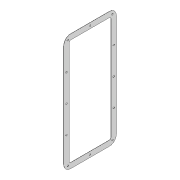
# Autodesk Inventor part: GB-gasket
Saved by Autodesk Inventor 2020 (Build 240168000, 168)
## iProperties
Created: 2021-06-24
Part Number: GB-gasket
Material: Generic
Document SubType Name: Modeling
Designer: Aidan Lee
Density: 1 g/cm^3
Appearance: Smooth - White
Author: Aidan Lee
Autodesk Inventor part; units mm, degrees
ref_plane "YZ Plane" through (0, 0, 0) normal (1, 0, 0) x (0, 1, 0)
ref_plane "XZ Plane" through (0, 0, 0) normal (0, 1, 0) x (-1, 0, 0)
ref_plane "XY Plane" through (0, 0, 0) normal (0, 0, 1) x (1, 0, 0)
sketch "Sketch1" plane through (0, 0, 0) normal (0, 0, 1) x (1, 0, 0)
  line L0 (0, 0) -> (140, 0) construction
  line L1 (140, 0) -> (140, 310) construction
  line L2 (140, 310) -> (0, 310) construction
  line L3 (0, 310) -> (0, 0) construction
  line L4 (15, 295) -> (125, 295) construction
  line L5 (125, 295) -> (125, 15) construction
  line L6 (125, 15) -> (15, 15) construction
  line L7 (15, 15) -> (15, 295) construction
  line L8 (15, 295) -> (125, 295) construction
  line L9 (70, 314.0975) -> (70, 322.6254) construction
  line L10 (15, 295) -> (15, 269.8596) construction
  line L11 (125, 295) -> (125, 292.6022) construction
  line L12 (0, 165.5) -> (-18, 165.5) construction
  line L13 (-18, 165.5) -> (-18, 185.5) construction
  line L14 (-18, 185.5) -> (0, 185.5) construction
  line L15 (0, 185.5) -> (0, 165.5) construction
  line L16 (-24.3067, 155) -> (-34.4998, 155) construction
  circle A0 centre (-9, 175.5) radius 3 construction
  line L17 (-18, 185.5) -> (0, 205.5) construction
  line L18 (0, 144.5) -> (-18, 144.5) construction
  line L19 (-18, 144.5) -> (-18, 124.5) construction
  circle A1 centre (-9, 134.5) radius 3 construction
  line L20 (-18, 124.5) -> (0, 104.5) construction
  line L21 (140, 165.5) -> (158, 165.5) construction
  line L22 (158, 165.5) -> (158, 185.5) construction
  circle A2 centre (149, 175.5) radius 3 construction
  line L23 (158, 185.5) -> (140, 205.5) construction
  line L24 (158, 144.5) -> (158, 124.5) construction
  line L25 (140, 144.5) -> (158, 144.5) construction
  circle A3 centre (149, 134.5) radius 3 construction
  line L26 (158, 124.5) -> (140, 104.5) construction
  line L27 (0, 300.2843) -> (9.7157, 310) construction
  line L28 (140, 300.2843) -> (130.2843, 310) construction
  line L29 (0, 9.7157) -> (9.7157, 0) construction
  line L30 (140, 9.7157) -> (130.2843, 0) construction
  line L31 (70, 295) -> (70, 310) construction
  line L32 (0, 155) -> (15, 155) construction
  line L33 (23.9173, 286.0827) -> (15, 295) construction
  line L34 (16.5096, 292.7523) -> (17.2477, 293.4904) construction
  line L35 (23.9173, 286.0827) -> (16.8787, 293.1213) construction
  line L36 (123.4904, 292.7523) -> (122.7523, 293.4904) construction
  line L37 (15, 17.2679) -> (15, 136.2679) construction
  arc A4 (14, 16.2679) -> (15, 17.2679) centre (14, 17.2679) ccw construction
  line L38 (14, 16.2679) -> (12, 16.2679) construction
  arc A5 (17, 17.2679) -> (18, 16.2679) centre (18, 17.2679) ccw construction
  spline S0 degree 3 poles (123.4904, 292.7523) (126.7806, 289.462) (122.6845, 284.0803) (122.5, 267.9145) knots 0 0 0 0 1 1 1 1 construction
  line L39 (15.2393, 288.9289) -> (15.2393, 218.384) construction
  line L40 (125, 148.5289) -> (125, 140.8711) construction
  line L41 (-110.1015, 148.4668) -> (-137.337, 121.2312) construction
  line L42 (-137.337, 121.2312) -> (-99.9418, 121.2312) construction
  line L43 (209.7417, 198.7679) -> (209.7417, 184.7679) construction
  line L44 (15, 148.5289) -> (15, 140.2675) construction
  line L45 (125, 148.5289) -> (125, 140.2675) construction
  spline S1 degree 4 poles (17.2477, 293.4904) (18.1955, 294.4381) (19.6714, 295.0826) (20.7017, 295) (21.8623, 295) knots 0 0 0 0 0 1 1 1 1 1 construction
  spline S2 degree 3 poles (122.7523, 293.4904) (121.4886, 294.7541) (119.4432, 295.1927) (118.1377, 295) knots 0 0 0 0 1 1 1 1 construction
  line L46 (118.1377, 295) -> (21.8623, 295) construction
  line L47 (16.8787, 293.1213) -> (23.2316, 286.7684) construction
  arc A6 (19, 310) -> (0, 291) centre (19, 291) ccw construction
  arc A7 (19, 295) -> (15, 291) centre (19, 291) ccw construction
  line L48 (19, 291) -> (10, 291) construction
  line L49 (19, 291) -> (19, 300) construction
  line L50 (16.1716, 293.8284) -> (5.565, 304.435) construction
  circle A8 centre (10.8683, 299.1317) radius 2 construction
  line L51 (9.8231, 300.915) -> (9.085, 300.1769) construction
  line L52 (11.9134, 297.3485) -> (12.6515, 298.0866) construction
  circle A9 centre (70, 302.5) radius 2 construction
  circle A10 centre (7.5, 155) radius 2 construction
  circle A11 centre (7.5, 227.0659) radius 2 construction
  line L53 (7.5, 155) -> (7.5, 227.0659) construction
  line L54 (7.5, 227.0659) -> (7.5, 299.1317) construction
  arc A12 (140, 291) -> (121, 310) centre (121, 291) ccw construction
  arc A13 (125, 291) -> (121, 295) centre (121, 291) ccw construction
  circle A14 centre (129.1317, 299.1317) radius 2 construction
  circle A15 centre (132.5, 155) radius 2 construction
  circle A16 centre (132.5, 227.0659) radius 2 construction
  circle A17 centre (10.8683, 10.8683) radius 2 construction
  circle A18 centre (70, 7.5) radius 2 construction
  circle A19 centre (7.5, 82.9341) radius 2 construction
  circle A20 centre (132.5, 82.9341) radius 2 construction
  circle A21 centre (129.1317, 10.8683) radius 2 construction
  arc A22 (0, 19) -> (19, 0) centre (19, 19) ccw construction
  arc A23 (15, 19) -> (19, 15) centre (19, 19) ccw construction
  arc A24 (121, 0) -> (140, 19) centre (121, 19) ccw construction
  arc A25 (121, 15) -> (125, 19) centre (121, 19) ccw construction
  circle A26 centre (10.8683, 299.1317) radius 7.5 construction
  line L55 (4.4716, 303.3416) -> (6.8718, 305.7419) construction
  line L56 (15, 140.2675) -> (15, 136.2679) construction
  line L57 (125, 138.6822) -> (125, 140.2675) construction
  line L58 (15, 138.6822) -> (15, 140.2675) construction
  line L59 (19, 15) -> (121, 15) construction
  line L60 (121, 0) -> (19, 0) construction
  line L61 (15, 291) -> (15, 19) construction
  line L62 (0, 19) -> (0, 291) construction
  line L63 (125, 291) -> (125, 19) construction
  line L64 (140, 19) -> (140, 291) construction
  line L65 (19, 295) -> (121, 295) construction
  line L66 (121, 310) -> (19, 310) construction
  arc A27 (132.5, 291) -> (121, 302.5) centre (121, 291) ccw construction
  arc A28 (139.5, 291) -> (121, 309.5) centre (121, 291) ccw
  arc A29 (125.5, 291) -> (121, 295.5) centre (121, 291) ccw
  arc A30 (125.5, 291) -> (139.5, 291) centre (132.5, 291) ccw construction
  arc A31 (121, 309.5) -> (121, 295.5) centre (121, 302.5) ccw construction
  arc A32 (19, 309.5) -> (0.5, 291) centre (19, 291) ccw
  arc A33 (19, 295.5) -> (14.5, 291) centre (19, 291) ccw
  arc A34 (121, 0.5) -> (139.5, 19) centre (121, 19) ccw
  arc A35 (121, 14.5) -> (125.5, 19) centre (121, 19) ccw
  arc A36 (14.5, 19) -> (19, 14.5) centre (19, 19) ccw
  arc A37 (0.5, 19) -> (19, 0.5) centre (19, 19) ccw
  line L67 (139.5, 19) -> (139.5, 291)
  line L68 (125.5, 291) -> (125.5, 19)
  line L69 (121, 14.5) -> (19, 14.5)
  line L70 (19, 0.5) -> (121, 0.5)
  line L71 (14.5, 19) -> (14.5, 291)
  line L72 (0.5, 291) -> (0.5, 19)
  line L73 (121, 295.5) -> (19, 295.5)
  line L74 (19, 309.5) -> (121, 309.5)
  point P0 (70, 318.3615)
  point P1 (-29.4032, 155)
  point P2 (-18, 175.5)
  point P3 (-9, 185.5)
  point P4 (124.7607, 288.9289)
  point P5 (209.7417, 191.7679)
  point P6 (19.6961, 294.835)
  point P7 (120.3039, 294.835)
  point P8 (9.4541, 300.5459)
  point P9 (12.2825, 297.7175)
  dimension "d163" = 4
  dimension "d0" = 140
  dimension "d1" = 310
  dimension "d2" = 15
  dimension "d85" = 18
  dimension "d86" = 20
  dimension "d87" = 10.5
  dimension "d88" = 6
  dimension "d89" = 20
  dimension "d114" = 135
  dimension "d126" = 1
  dimension "d128" = 2
  dimension "d152" = 45
  dimension "d158" = 45
  dimension "d161" = 4
  dimension "d164" = 5.5
  dimension "d168" = 15
  dimension "d169" = 1
  dimension "d170" = 1
  dimension "d171" = 1
  dimension "expansion" = 0.5
  dimension "d201" = 0.5
  constraints: 150 end point, 65 symmetric about line, 45 point on circle, 37 centre point, 16 midpoint, 16 parallel, 15 point on line, 14 tangent, 10 horizontal, 9 horizontal alignment, 9 vertical, 8 collinear, 8 perpendicular, 7 vertical alignment, 5 coincident, 3 equal length, 1 equal radius, 42 other
  measures "d0" distance of L0.start L0.end
  measures "d1" distance of L2.end L0.start
  measures "d2" distance between parallel lines of L2 L4
  measures "d85" distance of L13.end L14.end
  measures "d86" distance of L12.end L13.end
  measures "d87" distance between parallel lines of L12 L16
  measures "d88" diameter of A0
  measures "d89" vertical distance of L13.end L17.end
  measures "d114" angle of L3 L27
  measures "d126" radius of A4
  measures "d128" distance of L38.start L38.end
  measures "d152" angle of L42 L41
  measures "d158" angle of L4 L35
  measures "d161" radius of A7
  measures "d164" distance edge to line of A6 L51
  measures "d168" diameter of A26
  measures "d169" distance between parallel lines of L27 L55
  measures "d170" distance from line of L50.start L34
  measures "d171" horizontal distance between centres of A23 A5
  measures "expansion" radial gap between concentric circles of A12 A28
  measures "d201" radial gap between concentric circles of A13 A29
extrude "Extrusion7" add sketch "Sketch1" along normal blind 0.5
hole "Hole1" at (129.1317, 299.1317, 0) at (70, 302.5, 0) at (10.8683, 299.1317, 0) at (7.5, 227.0659, 0) at (132.5, 227.0659, 0) at (132.5, 155, 0) at (7.5, 155, 0) at (132.5, 82.9341, 0) at (129.1317, 10.8683, 0) at (70, 7.5, 0) at (10.8683, 10.8683, 0) at (7.5, 82.9341, 0) direction (0, 0, 1) diameter 4.1 end through all
body "Solid4"
